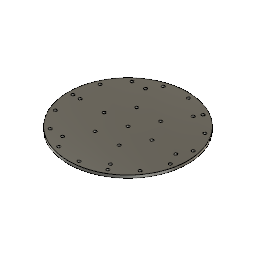
BASE_v1 v1 (Autodesk Fusion 360 design; units mm, degrees)
Autodesk Fusion 360 part; units mm, degrees
note: some values were not read from the file. Set by a fixed rule: which sketch regions a step uses.
sketch "Sketch1" plane through (0, 0, 0) normal (0, 0, 1) x (1, 0, 0)
  circle A0 centre (0, 0) radius 125
  line L0 (0, 0) -> (125, 0)
  line L1 (0, 0) -> (-62.5, -108.2532)
  line L2 (0, 0) -> (-62.5, 108.2532)
  line L3 (0, 0) -> (125, 0) construction
  line L4 (0, 0) -> (-25, 43.3013)
  line L5 (-25, 43.3013) -> (-50, 86.6025)
  line L6 (0, 0) -> (50, 0)
  line L7 (50, 0) -> (100, 0)
  line L8 (0, 0) -> (-25, -43.3013)
  line L9 (-25, -43.3013) -> (-50, -86.6025)
  circle A1 centre (-50, 86.6025) radius 3
  circle A2 centre (-25, 43.3013) radius 3
  circle A3 centre (50, 0) radius 3
  circle A4 centre (100, 0) radius 3
  circle A5 centre (-25, -43.3013) radius 3
  circle A6 centre (-50, -86.6025) radius 3
  line L10 (0, 0) -> (62.5, 108.2532)
  line L11 (0, 0) -> (125, 0) construction
  line L12 (0, 0) -> (62.5, -108.2532)
  line L13 (0, 0) -> (125, 0) construction
  line L14 (0, 0) -> (-125, 0)
  line L15 (0, 0) -> (-100, 0)
  circle A7 centre (-100, 0) radius 3
  line L16 (0, 0) -> (50, -86.6025)
  circle A8 centre (50, -86.6025) radius 3
  line L17 (0, 0) -> (50, 86.6025)
  circle A9 centre (50, 86.6025) radius 3
  circle A10 centre (0, 0) radius 3
  dimension "d1" = 250
  dimension "d2" = 60
  dimension "d3" = 120
  dimension "d4" = 50
  dimension "d5" = 50
  dimension "d6" = 50
  dimension "d7" = 50
  dimension "d8" = 50
  dimension "d9" = 50
  dimension "d10" = 6
  dimension "d11" = 6
  dimension "d12" = 6
  dimension "d13" = 6
  dimension "d14" = 6
  dimension "d15" = 6
  dimension "d16" = 60
  dimension "d17" = 60
  dimension "d18" = 100
  dimension "d19" = 6
  dimension "d20" = 100
  dimension "d21" = 6
  dimension "d22" = 100
  dimension "d23" = 6
  dimension "d24" = 6
  constraint coincident A0.centre L0.start
  constraint coincident A0 L0.end
  constraint horizontal L0
  constraint horizontal L3
  constraint parallel L2 L4
  constraint parallel L2 L5
  constraint parallel L3 L6
  constraint parallel L3 L7
  constraint parallel L1 L8
  constraint parallel L1 L9
  constraint coincident L5.end A1.centre
  constraint coincident L4.end L5.start
  constraint coincident L6.end L7.start
  constraint coincident L7.end A4.centre
  constraint coincident L8.end L9.start
  constraint coincident L9.end A6.centre
  constraint horizontal L11
  constraint horizontal L13
  constraint coincident A0 L14.end
  constraint horizontal L14
  constraint parallel L14 L15
  constraint coincident L15.end A7.centre
  constraint parallel L12 L16
  constraint coincident L16.end A8.centre
  constraint parallel L10 L17
  constraint coincident L17.end A9.centre
  measures "d1" diameter of A0
  measures "d2" angle of L0 L1
  measures "d3" angle of L2 L3
  measures "d4" distance of A0.centre L4.end
  measures "d5" distance of L4.end L5.end
  measures "d6" distance of A0.centre L6.end
  measures "d7" distance of L6.end L7.end
  measures "d8" distance of A0.centre L8.end
  measures "d9" distance of L8.end L9.end
  measures "d10" diameter of A1
  measures "d11" diameter of A2
  measures "d12" diameter of A3
  measures "d13" diameter of A4
  measures "d14" diameter of A5
  measures "d15" diameter of A6
  measures "d16" angle of L10 L11
  measures "d17" angle of L12 L13
  measures "d18" distance of A0.centre L15.end
  measures "d19" diameter of A7
  measures "d20" distance of A0.centre L16.end
  measures "d21" diameter of A8
  measures "d22" distance of A0.centre L17.end
  measures "d23" diameter of A9
  measures "d24" diameter of A10
extrude "Extrude1" add sketch "Sketch1" along normal blind 6 contours A0 L0 L6 L7 A3 A4 L10 L17 A9 A10 | A0 L0 L6 L7 A3 A4 L12 L16 A8 A10 | A0 L2 L4 L5 A1 A2 L10 L17 A9 A10 | A0 L1 L8 L9 A5 A6 L12 L16 A8 A10 | A0 L2 L4 L5 A1 A2 L14 L15 A7 A10 | A0 L1 L8 L9 A5 A6 L14 L15 A7 A10
sketch "Sketch2" plane through (0, 0, 6) normal (0, 0, 1) x (-1, 0, 0)
  circle A0 centre (0, 0) radius 3
  circle A1 centre (-50, -86.6025) radius 3
  circle A2 centre (25, -43.3013) radius 3
  circle A3 centre (100, 0) radius 3
  circle A4 centre (25, 43.3013) radius 3
  circle A5 centre (50, -86.6025) radius 3
  circle A6 centre (-100, 0) radius 3
  circle A7 centre (-50, 86.6025) radius 3
  circle A8 centre (-50, 0) radius 3
  circle A9 centre (50, 86.6025) radius 3
  circle A10 centre (0, 0) radius 125
  line L0 (125, 0) -> (115, 0)
  circle A11 centre (115, 0) radius 3
  circle A12 centre (105.0577, 46.7747) radius 3
  circle A13 centre (76.95, 85.4617) radius 3
  circle A14 centre (35.537, 109.3715) radius 3
  circle A15 centre (-12.0208, 114.37) radius 3
  circle A16 centre (-57.5, 99.5929) radius 3
  circle A17 centre (-93.037, 67.5953) radius 3
  circle A18 centre (-112.487, 23.9098) radius 3
  circle A19 centre (-112.487, -23.9098) radius 3
  circle A20 centre (-93.037, -67.5953) radius 3
  circle A21 centre (-57.5, -99.5929) radius 3
  circle A22 centre (-12.0208, -114.37) radius 3
  circle A23 centre (35.537, -109.3715) radius 3
  circle A24 centre (76.95, -85.4617) radius 3
  circle A25 centre (105.0577, -46.7747) radius 3
  dimension "d27" = 10
  dimension "d28" = 6
  dimension "d30" = 360
  constraint coincident A10 L0.start
  constraint horizontal L0
  constraint coincident L0.end A11.centre
  measures "d27" distance of L0.start L0.end
  measures "d28" diameter of A11
extrude "Extrude2" cut sketch "Sketch2" against normal blind 6 contours A11 | A12 | A13 | A14 | A15 | A16 | A17 | A18 | A19 | A20 | A21 | A22 | A23 | A24 | A25
sketch "Sketch3" plane through (0, 0, 6) normal (0, 0, 1) x (-1, 0, 0)
  circle A0 centre (35.537, 109.3715) radius 3
  circle A1 centre (-112.487, 23.9098) radius 3
  circle A2 centre (-12.0208, -114.37) radius 3
  circle A3 centre (115, 0) radius 3
  circle A4 centre (35.537, -109.3715) radius 3
  circle A5 centre (-112.487, -23.9098) radius 3
  circle A6 centre (-12.0208, 114.37) radius 3
  circle A7 centre (76.95, 85.4617) radius 3
  circle A8 centre (-93.037, 67.5953) radius 3
  circle A9 centre (-57.5, -99.5929) radius 3
  circle A10 centre (105.0577, -46.7747) radius 3
  circle A11 centre (76.95, -85.4617) radius 3
  circle A12 centre (-93.037, -67.5953) radius 3
  circle A13 centre (-57.5, 99.5929) radius 3
  circle A14 centre (105.0577, 46.7747) radius 3
  circle A15 centre (0, 0) radius 3
  circle A16 centre (-50, -86.6025) radius 3
  circle A17 centre (25, -43.3013) radius 3
  circle A18 centre (100, 0) radius 3
  circle A19 centre (25, 43.3013) radius 3
  circle A20 centre (50, -86.6025) radius 3
  circle A21 centre (-100, 0) radius 3
  circle A22 centre (-50, 86.6025) radius 3
  circle A23 centre (-50, 0) radius 3
  circle A24 centre (50, 86.6025) radius 3
  circle A25 centre (0, 0) radius 125
  line L0 (0, 0) -> (50, 0)
  line L1 (0, 0) -> (-50, -86.6025)
  line L2 (-50, 86.6025) -> (0, 0)
  circle A26 centre (-25, -43.3013) radius 3
  circle A27 centre (-25, 43.3013) radius 3
  circle A28 centre (50, 0) radius 3
  dimension "d33" = 50
  dimension "d34" = 6
  dimension "d35" = 6
  dimension "d36" = 6
  constraint coincident A15.centre A25.centre
  constraint horizontal L0
  constraint coincident A16.centre L1.end
  constraint coincident A22.centre L2.start
  constraint midpoint L1 A26.centre
  constraint midpoint L2 A27.centre
  constraint coincident L0.end A28.centre
  measures "d33" distance of A15.centre L0.end
  measures "d34" diameter of A26
  measures "d35" diameter of A27
  measures "d36" diameter of A28
extrude "Extrude3" cut sketch "Sketch3" against normal blind 6 contours L1 A26 | L1 A26 | L2 A27 | L2 A27 | A28
